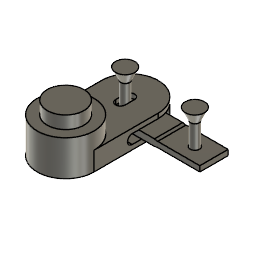
Kurbelschleife (Autodesk Fusion 360 design; units mm, degrees)
Autodesk Fusion 360 part; units mm, degrees
note: some values were not read from the file. Set by a fixed rule: which face or edge a step refers to.
box "Grundkörper Quader1" add length 32 width 15 height 5 placed x (0, 1, 0) y (-1, 0, 0) z (0, 0, 1) at (20, 0, 0) makes body 1
fillet "Abrundung1" radius 7.5 4 edges at (20, 0, 2.5) (5, 0, 2.5) (20, 32, 2.5) (5, 32, 2.5) on bodies 1
sketch "Skizze2" plane through (0, 0, 5) normal (0, 0, 1) x (-1, 0, 0)
  arc A0 (-20, -24.5) -> (-5, -24.5) centre (-12.5, -24.5) ccw
  line L0 (-5, -24.5) -> (-5, -7.5)
  arc A1 (-5, -7.5) -> (-20, -7.5) centre (-12.5, -7.5) ccw
  line L1 (-20, -7.5) -> (-20, -24.5)
  circle A2 centre (-12.5, -7.5) radius 5
  line L2 (-11.25, -24.5) -> (-11.25, -22)
  arc A3 (-11.25, -22) -> (-13.75, -22) centre (-12.5, -22) ccw
  line L3 (-13.75, -22) -> (-13.75, -24.5)
  arc A4 (-13.75, -24.5) -> (-11.25, -24.5) centre (-12.5, -24.5) ccw
  line L4 (-12.5, -24.5) -> (-12.5, -22) construction
  circle A5 centre (-12.5, -23.25) radius 1.25
  dimension "d8" = 10
  dimension "d11" = 2.5
  dimension "d12" = 2.5
  dimension "d13" = 1.25
  constraint concentric A1 A2
  constraint tangent L2 A3
  constraint tangent A3 L3
  constraint parallel L2 L3
  constraint tangent L3 A4
  constraint tangent L2 A4
  constraint parallel L0 L4
  constraint coincident A0.centre A4.centre
  constraint midpoint L4 A5.centre
  measures "d8" diameter of A2
  measures "d11" diameter of A5
  measures "d12" distance of A0.centre A3.centre
  measures "d13" radius of A3
extrude "Extrusion1" cut sketch "Skizze2" against normal blind 10 contours A2 | L2 L3 A4 A5 | L2 A3 L3 A5 | A5 bodies 1
extrude "Extrusion2" add sketch "Skizze2" against normal blind 10 separate body contours A5 makes body 2
sketch "Skizze4" plane through (20, 0, 0) normal (1, 0, 0) x (0, 1, 0)
  line L0 (24.5, 0) -> (24.5, 5)
  line L1 (24.5, 5) -> (7.5, 5)
  line L2 (7.5, 5) -> (7.5, 0)
  line L3 (7.5, 0) -> (24.5, 0)
  line L4 (17.625, 1.25) -> (28.875, 1.25)
  arc A0 (28.875, 1.25) -> (28.875, 3.75) centre (28.875, 2.5) ccw
  line L5 (28.875, 3.75) -> (17.625, 3.75)
  arc A1 (17.625, 3.75) -> (17.625, 1.25) centre (17.625, 2.5) ccw
  line L6 (17.625, 2.5) -> (28.875, 2.5) construction
  dimension "d25" = 2.5
  dimension "d63" = 11.25
  dimension "d66" = 1.25
  dimension "d67" = 1.25
  dimension "d70" = 6.875
  constraint tangent L4 A0
  constraint tangent A0 L5
  constraint parallel L4 L5
  constraint tangent L5 A1
  constraint tangent L4 A1
  constraint perpendicular L0 L6
  measures "d25" diameter of A0
  measures "d63" distance of A1.centre A0.centre
  measures "d66" distance of L1 L5
  measures "d67" distance of L3 L4
  measures "d70" distance of L0 A1.centre
extrude "Extrusion3" cut sketch "Skizze4" against normal blind 15 contours L0 L4 L5 A1 | L0 L4 A0 L5 bodies 1
sketch "Skizze5" plane through (0, 0, 5) normal (0, 0, 1) x (-1, 0, 0)
  line L0 (-5, -24.5) -> (-5, -7.5)
  arc A0 (-5, -7.5) -> (-20, -7.5) centre (-12.5, -7.5) ccw
  line L1 (-20, -7.5) -> (-20, -24.5)
  line L2 (-9, -27, -1.3919) -> (-24, -27, -1.3919)
  line L3 (-24, -27, -1.3919) -> (-24, -19.5, -1.3919)
  line L4 (-24, -19.5, -1.3919) -> (-9, -19.5, -1.3919)
  line L5 (-9, -19.5, -1.3919) -> (-9, -27, -1.3919)
  arc A1 (-11.25, -22) -> (-13.75, -22) centre (-12.5, -22) ccw
  line L6 (-11.25, -22) -> (-11.25, -24.5)
  arc A2 (-13.75, -24.5) -> (-11.25, -24.5) centre (-12.5, -24.5) ccw
  line L7 (-13.75, -24.5) -> (-13.75, -22)
  arc A3 (-20, -24.5) -> (-5, -24.5) centre (-12.5, -24.5) ccw
  circle A4 centre (-12.5, -7.5) radius 5
  circle A5 centre (-12.5, -23.25) radius 1.25
  dimension "d28" = 15
  dimension "d29" = 7.5
extrude "Extrusion4" add sketch "Skizze5" against normal blind 1.75 separate body contours L2 L3 L4 L5 in plane through (0, 0, 3.6081) normal (0, 0, 1) makes body 3
fillet "Abrundung2" radius 3.75 2 edges at (9, 19.5, 2.7331) (9, 27, 2.7331) on bodies 3
extrude "Extrusion5" cut sketch "Skizze2" against normal blind 5 contours A5 bodies 3
sketch "Skizze6" plane through (24, 0, 0) normal (1, 0, 0) x (0, 1, 0)
  line L0 (27, 3.6081) -> (19.5, 3.6081)
  line L1 (19.5, 3.6081) -> (19.5, 1.8581)
  line L2 (19.5, 1.8581) -> (27, 1.8581)
  line L3 (27, 1.8581) -> (27, 3.6081)
  line L4 (19.5, 3.4581) -> (27, 3.4581)
  line L5 (27, 3.4581) -> (27, 2.0081)
  line L6 (27, 2.0081) -> (19.5, 2.0081)
  line L7 (19.5, 2.0081) -> (19.5, 3.4581)
  dimension "d42" = 0.15
  dimension "d43" = 1.45
  constraint horizontal L4
  constraint vertical L5
  constraint horizontal L6
  constraint vertical L7
  constraint coincident L3 L5.end
  constraint coincident L1 L4.start
  measures "d42" distance of L0 L4
  measures "d43" distance of L4.end L5.end
extrude "Extrusion6" add sketch "Skizze6" along normal blind 12 contours L1 L3 L4 L5 L6 L7 bodies 3
fillet "Abrundung3" radius 2.5 2 edges at (24, 23.25, 3.4581) (24, 23.25, 2.0081) on bodies 3
sketch "Skizze7" plane through (0, 0, 3.4581) normal (0, 0, 1) x (-1, 0, 0)
  line L0 (-24.8529, -19.5) -> (-36, -19.5)
  line L1 (-36, -19.5) -> (-36, -27)
  line L2 (-36, -27) -> (-24.8529, -27)
  circle A0 centre (-30.94, -23.25) radius 1.25
  line L3 (-24.8529, -27) -> (-24.8529, -19.5)
  dimension "d48" = 2.5
  dimension "d57" = 5.06
  dimension "d64" = 3.75
  dimension "d65" = 3.75
  measures "d48" diameter of A0
  measures "d57" distance of L1 A0.centre
  measures "d64" distance of L2 A0.centre
  measures "d65" distance of L0 A0.centre
extrude "Extrusion7" cut sketch "Skizze7" against normal blind 1.45 contours A0 bodies 3
extrude "Extrusion8" add sketch "Skizze7" along normal blind 10 separate body contours A0 makes body 4
move_face "Flächen versetzen2" offset -0.1 3 faces at (11.2516, 23.3123, -1.6667) (13.6746, 22.8225, -1.6667) (29.6916, 23.3123, 10.1247) on bodies 2 4
move_body "Verschieben1" bodies 4 to x (1, 0, 0) y (0, 1, 0) z (0, 0, 1) at (0, 0, -4)
sketch "Skizze8" plane through (0, 0, 0) normal (0, 0, -1) x (1, 0, 0)
  line L0 (11.25, -24.5) -> (11.25, -22)
  arc A0 (13.75, -22) -> (11.25, -22) centre (12.5, -22) ccw
  line L1 (13.75, -22) -> (13.75, -24.5)
  arc A1 (11.25, -24.5) -> (13.75, -24.5) centre (12.5, -24.5) ccw
  circle A2 centre (12.5, -7.5) radius 5
  arc A3 (5, -24.5) -> (20, -24.5) centre (12.5, -24.5) ccw
  line L2 (20, -24.5) -> (20, -7.5)
  arc A4 (20, -7.5) -> (5, -7.5) centre (12.5, -7.5) ccw
  line L3 (5, -7.5) -> (5, -24.5)
extrude "Extrusion9" add sketch "Skizze8" against normal blind 12.75 contours A2 bodies 1
move_face "Flächen versetzen3" offset -0.15 1 faces at (17.4752, 7.0022, 7.5833) on bodies 1
cylinder "Grundkörper Zylinder1" add diameter 15 height 4.4 placed x (1, 0, 0) y (0, 1, 0) z (0, 0, 1) at (12.5, 7.5, 5) bodies 1
move_body "Verschieben2" bodies 2 to x (1, 0, 0) y (0, 1, 0) z (0, 0, 1) at (0, 0, 4.4581)
extrude "Extrusion11" add 2 faces at (12.5834, 22.9017, 9.4581) (30.7256, 23.2948, 9.4581) along direction (0, 0, 1) blind 3 draft 25 on bodies 2 4 bodies 2 4
equation "d1 = Basis_X"
equation "d2 = Basis_Y"
equation "d3 = Basis_Z"
equation "d7 = Abrundung"
equation "d8 = Loch_Durchmesser"
equation "d9 = Loch_Tiefe"
equation "d11 = Langloch_Stick"
equation "d12 = Langloch_Länge"
equation "d13 = Langloch_Radius"
equation "Basis_X = 32 mm"
equation "Basis_Y = 15 mm"
equation "Basis_Z = 5 mm"
equation "Abrundung = Basis_Y / 2"
equation "Loch_Tiefe = -Basis_Z * 2"
equation "d19 = Loch_Tiefe"
equation "Langloch_Länge = 2.5 mm"
equation "Loch_Durchmesser = 10 mm"
equation "Langloch_Radius = 1.25 mm"
equation "Langloch_Stick = Langloch_Radius * 2"
equation "d25 = Langloch_Radius * 2"
equation "d26 = -Basis_Y"
equation "d28 = Schieber_Länge"
equation "d29 = Schieber_Breite"
equation "Versatz = 0.05 mm"
equation "Schieber_Länge = 15 mm"
equation "Schieber_Breite = 7.5 mm"
equation "Schieber_Höhe = -2.25 mm + Versatz * 10"
equation "d34 = Schieber_Höhe"
equation "d37 = Schieber_Abrundung"
equation "d38 = -Basis_Z"
equation "d42 = Halter_Abstand_Innen"
equation "d43 = Halter_Höhe"
equation "d44 = Halter_Länge"
equation "d47 = Abrundung_Verbindung"
equation "d48 = Loch_Halter"
equation "d49 = -Halter_Höhe"
equation "Halter_Höhe = 1.45 mm"
equation "Halter_Abstand_Innen = ( -Schieber_Höhe - Halter_Höhe ) / 2"
equation "Schieber_Abrundung = Schieber_Breite / 2"
equation "Halter_Länge = 12 mm"
equation "Abrundung_Verbindung = 2.5 mm"
equation "Loch_Halter = 2.5 mm"
equation "d57 = Loch_Abstand"
equation "Loch_Abstand = 5.06 mm"
equation "d59 = Halter_Stick"
equation "d61 = -Versatz * 2"
equation "Halter_Stick = 10 mm"
equation "d63 = Langloch_Länge_Seite"
equation "d64 = Schieber_Breite / 2"
equation "d66 = Basis_Z / 4"
equation "d70 = Langloch_Länge_Abstand"
equation "Langloch_Länge_Seite = 11.25 mm"
equation "Langloch_Länge_Abstand = 6.875 mm"
